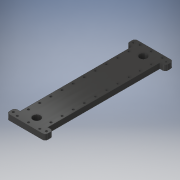
# Autodesk Inventor part: PVCBottom
Saved by Autodesk Inventor 2019.4 (Build 234330000, 330)
## iProperties
Created: 2020-04-27
Part Number: PVCBottom
Material: Generic
Document SubType Name: Modeling
Designer: Ed
Density: 1 g/cm^3
Appearance: Default
Author: Ed
Autodesk Inventor part; units mm, degrees
ref_plane "YZ Plane" through (0, 0, 0) normal (1, 0, 0) x (0, 1, 0)
ref_plane "XZ Plane" through (0, 0, 0) normal (0, 1, 0) x (-1, 0, 0)
ref_plane "XY Plane" through (0, 0, 0) normal (0, 0, 1) x (1, 0, 0)
sketch "Sketch1" plane through (0, 0, 0) normal (0, 1, 0) x (-1, 0, 0)
  line L0 (50.8, 0) -> (52.1295, 0)
  arc A0 (50.8, 16.637) -> (59.7281, 25.5651) centre (50.8, 25.5651) ccw
  arc A1 (59.7281, 25.5651) -> (50.8, 34.4932) centre (50.8, 25.5651) ccw
  arc A2 (50.8, 34.4932) -> (41.8719, 25.5651) centre (50.8, 25.5651) ccw
  arc A3 (41.8719, 25.5651) -> (50.8, 16.637) centre (50.8, 25.5651) ccw
  arc A4 (53.213, 6.35) -> (50.721, 8.7617) centre (50.8, 6.35) ccw
  arc A5 (50.721, 8.7617) -> (50.1755, 8.6808) centre (50.8, 6.35) ccw
  arc A6 (50.1755, 8.6808) -> (48.387, 6.35) centre (50.8, 6.35) ccw
  arc A7 (48.387, 6.35) -> (53.1308, 5.7255) centre (50.8, 6.35) ccw
  arc A8 (53.1308, 5.7255) -> (53.1924, 6.035) centre (50.8, 6.35) ccw
  arc A9 (53.1924, 6.035) -> (53.2078, 6.1922) centre (50.8, 6.35) ccw
  arc A10 (53.2078, 6.1922) -> (53.213, 6.35) centre (50.8, 6.35) ccw
  arc A11 (87.6788, 9.0295) -> (87.7165, 8.8676) centre (90.17, 9.525) ccw
  arc A12 (87.7165, 8.8676) -> (92.71, 9.525) centre (90.17, 9.525) ccw
  arc A13 (92.71, 9.525) -> (87.63, 9.525) centre (90.17, 9.525) ccw
  arc A14 (87.63, 9.525) -> (87.6788, 9.0295) centre (90.17, 9.525) ccw
  arc A15 (77.5292, 8.7623) -> (76.8455, 8.6808) centre (77.47, 6.35) ccw
  arc A16 (76.8455, 8.6808) -> (75.057, 6.35) centre (77.47, 6.35) ccw
  arc A17 (75.057, 6.35) -> (79.883, 6.35) centre (77.47, 6.35) ccw
  arc A18 (79.883, 6.35) -> (79.3353, 7.8808) centre (77.47, 6.35) ccw
  arc A19 (79.3353, 7.8808) -> (77.5292, 8.7623) centre (77.47, 6.35) ccw
  arc A20 (77.6672, 35.3094) -> (76.8455, 35.2352) centre (77.47, 32.9044) ccw
  arc A21 (76.8455, 35.2352) -> (75.057, 32.9044) centre (77.47, 32.9044) ccw
  arc A22 (75.057, 32.9044) -> (77.6278, 30.4966) centre (77.47, 32.9044) ccw
  arc A23 (77.6278, 30.4966) -> (79.5597, 31.6979) centre (77.47, 32.9044) ccw
  arc A24 (79.5597, 31.6979) -> (79.883, 32.9044) centre (77.47, 32.9044) ccw
  arc A25 (79.883, 32.9044) -> (77.9408, 35.2711) centre (77.47, 32.9044) ccw
  arc A26 (77.9408, 35.2711) -> (77.6672, 35.3094) centre (77.47, 32.9044) ccw
  arc A27 (77.5292, 61.8711) -> (76.8455, 61.7896) centre (77.47, 59.4589) ccw
  arc A28 (76.8455, 61.7896) -> (75.057, 59.4589) centre (77.47, 59.4589) ccw
  arc A29 (75.057, 59.4589) -> (76.8455, 57.1281) centre (77.47, 59.4589) ccw
  arc A30 (76.8455, 57.1281) -> (77.391, 57.0472) centre (77.47, 59.4589) ccw
  arc A31 (77.391, 57.0472) -> (79.883, 59.4589) centre (77.47, 59.4589) ccw
  arc A32 (79.883, 59.4589) -> (79.3353, 60.9897) centre (77.47, 59.4589) ccw
  arc A33 (79.3353, 60.9897) -> (77.5292, 61.8711) centre (77.47, 59.4589) ccw
  arc A34 (77.6672, 88.4182) -> (76.8455, 88.3441) centre (77.47, 86.0133) ccw
  arc A35 (76.8455, 88.3441) -> (75.057, 86.0133) centre (77.47, 86.0133) ccw
  arc A36 (75.057, 86.0133) -> (77.6278, 83.6055) centre (77.47, 86.0133) ccw
  arc A37 (77.6278, 83.6055) -> (79.5597, 84.8068) centre (77.47, 86.0133) ccw
  arc A38 (79.5597, 84.8068) -> (79.883, 86.0133) centre (77.47, 86.0133) ccw
  arc A39 (79.883, 86.0133) -> (77.9408, 88.3799) centre (77.47, 86.0133) ccw
  arc A40 (77.9408, 88.3799) -> (77.6672, 88.4182) centre (77.47, 86.0133) ccw
  arc A41 (77.6672, 114.9726) -> (76.8455, 114.8985) centre (77.47, 112.5677) ccw
  arc A42 (76.8455, 114.8985) -> (75.057, 112.5677) centre (77.47, 112.5677) ccw
  arc A43 (75.057, 112.5677) -> (76.8455, 110.2369) centre (77.47, 112.5677) ccw
  arc A44 (76.8455, 110.2369) -> (77.391, 110.156) centre (77.47, 112.5677) ccw
  arc A45 (77.391, 110.156) -> (79.883, 112.5677) centre (77.47, 112.5677) ccw
  arc A46 (79.883, 112.5677) -> (79.6342, 113.635) centre (77.47, 112.5677) ccw
  arc A47 (79.6342, 113.635) -> (77.6672, 114.9726) centre (77.47, 112.5677) ccw
  arc A48 (77.6278, 141.53) -> (76.2635, 141.2119) centre (77.47, 139.1222) ccw
  arc A49 (76.2635, 141.2119) -> (75.057, 139.1222) centre (77.47, 139.1222) ccw
  arc A50 (75.057, 139.1222) -> (77.2335, 136.7208) centre (77.47, 139.1222) ccw
  arc A51 (77.2335, 136.7208) -> (79.1762, 137.4159) centre (77.47, 139.1222) ccw
  arc A52 (79.1762, 137.4159) -> (79.883, 139.1222) centre (77.47, 139.1222) ccw
  arc A53 (79.883, 139.1222) -> (78.0945, 141.4529) centre (77.47, 139.1222) ccw
  arc A54 (78.0945, 141.4529) -> (77.6278, 141.53) centre (77.47, 139.1222) ccw
  arc A55 (77.6278, 168.0844) -> (76.2635, 167.7663) centre (77.47, 165.6766) ccw
  arc A56 (76.2635, 167.7663) -> (75.057, 165.6766) centre (77.47, 165.6766) ccw
  arc A57 (75.057, 165.6766) -> (76.8455, 163.3458) centre (77.47, 165.6766) ccw
  arc A58 (76.8455, 163.3458) -> (77.391, 163.2649) centre (77.47, 165.6766) ccw
  arc A59 (77.391, 163.2649) -> (79.883, 165.6766) centre (77.47, 165.6766) ccw
  arc A60 (79.883, 165.6766) -> (79.5597, 166.8831) centre (77.47, 165.6766) ccw
  arc A61 (79.5597, 166.8831) -> (77.6278, 168.0844) centre (77.47, 165.6766) ccw
  arc A62 (77.6278, 194.6388) -> (76.2635, 194.3207) centre (77.47, 192.231) ccw
  arc A63 (76.2635, 194.3207) -> (75.057, 192.231) centre (77.47, 192.231) ccw
  arc A64 (75.057, 192.231) -> (77.2335, 189.8296) centre (77.47, 192.231) ccw
  arc A65 (77.2335, 189.8296) -> (79.1762, 190.5248) centre (77.47, 192.231) ccw
  arc A66 (79.1762, 190.5248) -> (79.883, 192.231) centre (77.47, 192.231) ccw
  arc A67 (79.883, 192.231) -> (78.0945, 194.5618) centre (77.47, 192.231) ccw
  arc A68 (78.0945, 194.5618) -> (77.6278, 194.6388) centre (77.47, 192.231) ccw
  arc A69 (77.5958, 221.1952) -> (77.4404, 221.1983) centre (77.47, 218.7854) ccw
  arc A70 (77.4404, 221.1983) -> (75.7638, 220.4917) centre (77.47, 218.7854) ccw
  arc A71 (75.7638, 220.4917) -> (75.057, 218.7854) centre (77.47, 218.7854) ccw
  arc A72 (75.057, 218.7854) -> (76.8455, 216.4547) centre (77.47, 218.7854) ccw
  arc A73 (76.8455, 216.4547) -> (77.391, 216.3737) centre (77.47, 218.7854) ccw
  arc A74 (77.391, 216.3737) -> (79.883, 218.7854) centre (77.47, 218.7854) ccw
  arc A75 (79.883, 218.7854) -> (79.7791, 219.4859) centre (77.47, 218.7854) ccw
  arc A76 (79.7791, 219.4859) -> (78.0563, 221.1261) centre (77.47, 218.7854) ccw
  arc A77 (78.0563, 221.1261) -> (77.5958, 221.1952) centre (77.47, 218.7854) ccw
  arc A78 (77.7065, 247.7413) -> (75.7638, 247.0461) centre (77.47, 245.3399) ccw
  arc A79 (75.7638, 247.0461) -> (75.057, 245.3399) centre (77.47, 245.3399) ccw
  arc A80 (75.057, 245.3399) -> (77.2335, 242.9385) centre (77.47, 245.3399) ccw
  arc A81 (77.2335, 242.9385) -> (79.1762, 243.6336) centre (77.47, 245.3399) ccw
  arc A82 (79.1762, 243.6336) -> (79.883, 245.3399) centre (77.47, 245.3399) ccw
  arc A83 (79.883, 245.3399) -> (77.7065, 247.7413) centre (77.47, 245.3399) ccw
  arc A84 (76.8455, 269.5635) -> (77.391, 269.4826) centre (77.47, 271.8943) ccw
  arc A85 (77.391, 269.4826) -> (79.883, 271.8943) centre (77.47, 271.8943) ccw
  arc A86 (79.883, 271.8943) -> (79.7283, 272.7443) centre (77.47, 271.8943) ccw
  arc A87 (79.7283, 272.7443) -> (78.1041, 274.2225) centre (77.47, 271.8943) ccw
  arc A88 (78.1041, 274.2225) -> (77.6364, 274.3016) centre (77.47, 271.8943) ccw
  arc A89 (77.6364, 274.3016) -> (75.1392, 272.5188) centre (77.47, 271.8943) ccw
  arc A90 (75.1392, 272.5188) -> (75.057, 271.8943) centre (77.47, 271.8943) ccw
  arc A91 (75.057, 271.8943) -> (76.8455, 269.5635) centre (77.47, 271.8943) ccw
  arc A92 (13.8835, 8.8676) -> (13.97, 9.525) centre (11.43, 9.525) ccw
  arc A93 (13.97, 9.525) -> (8.89, 9.525) centre (11.43, 9.525) ccw
  arc A94 (8.89, 9.525) -> (13.8835, 8.8676) centre (11.43, 9.525) ccw
  arc A95 (24.13, 8.763) -> (22.7894, 8.3563) centre (24.13, 6.35) ccw
  arc A96 (22.7894, 8.3563) -> (21.717, 6.35) centre (24.13, 6.35) ccw
  arc A97 (21.717, 6.35) -> (26.4608, 5.7255) centre (24.13, 6.35) ccw
  arc A98 (26.4608, 5.7255) -> (26.543, 6.35) centre (24.13, 6.35) ccw
  arc A99 (26.543, 6.35) -> (26.3593, 7.2734) centre (24.13, 6.35) ccw
  arc A100 (26.3593, 7.2734) -> (24.13, 8.763) centre (24.13, 6.35) ccw
  arc A101 (24.2632, 35.3138) -> (24.13, 35.3174) centre (24.13, 32.9044) ccw
  arc A102 (24.13, 35.3174) -> (21.717, 32.9044) centre (24.13, 32.9044) ccw
  arc A103 (21.717, 32.9044) -> (22.7894, 30.8981) centre (24.13, 32.9044) ccw
  arc A104 (22.7894, 30.8981) -> (23.5055, 30.5737) centre (24.13, 32.9044) ccw
  arc A105 (23.5055, 30.5737) -> (24.051, 30.4927) centre (24.13, 32.9044) ccw
  arc A106 (24.051, 30.4927) -> (26.543, 32.9044) centre (24.13, 32.9044) ccw
  arc A107 (26.543, 32.9044) -> (24.6008, 35.2711) centre (24.13, 32.9044) ccw
  arc A108 (24.6008, 35.2711) -> (24.4841, 35.2913) centre (24.13, 32.9044) ccw
  arc A109 (24.4841, 35.2913) -> (24.3075, 35.3109) centre (24.13, 32.9044) ccw
  arc A110 (24.3075, 35.3109) -> (24.2632, 35.3138) centre (24.13, 32.9044) ccw
  arc A111 (24.13, 61.8719) -> (22.7894, 61.4652) centre (24.13, 59.4589) ccw
  arc A112 (22.7894, 61.4652) -> (21.717, 59.4589) centre (24.13, 59.4589) ccw
  arc A113 (21.717, 59.4589) -> (23.5055, 57.1281) centre (24.13, 59.4589) ccw
  arc A114 (23.5055, 57.1281) -> (24.051, 57.0472) centre (24.13, 59.4589) ccw
  arc A115 (24.051, 57.0472) -> (26.543, 59.4589) centre (24.13, 59.4589) ccw
  arc A116 (26.543, 59.4589) -> (24.13, 61.8719) centre (24.13, 59.4589) ccw
  arc A117 (24.2632, 88.4226) -> (24.13, 88.4263) centre (24.13, 86.0133) ccw
  arc A118 (24.13, 88.4263) -> (21.717, 86.0133) centre (24.13, 86.0133) ccw
  arc A119 (21.717, 86.0133) -> (23.5055, 83.6825) centre (24.13, 86.0133) ccw
  arc A120 (23.5055, 83.6825) -> (24.051, 83.6016) centre (24.13, 86.0133) ccw
  arc A121 (24.051, 83.6016) -> (26.543, 86.0133) centre (24.13, 86.0133) ccw
  arc A122 (26.543, 86.0133) -> (24.6008, 88.3799) centre (24.13, 86.0133) ccw
  arc A123 (24.6008, 88.3799) -> (24.4841, 88.4002) centre (24.13, 86.0133) ccw
  arc A124 (24.4841, 88.4002) -> (24.3075, 88.4198) centre (24.13, 86.0133) ccw
  arc A125 (24.3075, 88.4198) -> (24.2632, 88.4226) centre (24.13, 86.0133) ccw
  arc A126 (24.13, 114.9807) -> (22.4238, 114.274) centre (24.13, 112.5677) ccw
  arc A127 (22.4238, 114.274) -> (21.717, 112.5677) centre (24.13, 112.5677) ccw
  arc A128 (21.717, 112.5677) -> (23.5055, 110.2369) centre (24.13, 112.5677) ccw
  arc A129 (23.5055, 110.2369) -> (24.051, 110.156) centre (24.13, 112.5677) ccw
  arc A130 (24.051, 110.156) -> (26.543, 112.5677) centre (24.13, 112.5677) ccw
  arc A131 (26.543, 112.5677) -> (24.13, 114.9807) centre (24.13, 112.5677) ccw
  arc A132 (24.2632, 141.5315) -> (24.13, 141.5352) centre (24.13, 139.1222) ccw
  arc A133 (24.13, 141.5352) -> (21.717, 139.1222) centre (24.13, 139.1222) ccw
  arc A134 (21.717, 139.1222) -> (23.5055, 136.7914) centre (24.13, 139.1222) ccw
  arc A135 (23.5055, 136.7914) -> (24.051, 136.7104) centre (24.13, 139.1222) ccw
  arc A136 (24.051, 136.7104) -> (26.543, 139.1222) centre (24.13, 139.1222) ccw
  arc A137 (26.543, 139.1222) -> (24.6008, 141.4888) centre (24.13, 139.1222) ccw
  arc A138 (24.6008, 141.4888) -> (24.4841, 141.509) centre (24.13, 139.1222) ccw
  arc A139 (24.4841, 141.509) -> (24.3075, 141.5286) centre (24.13, 139.1222) ccw
  arc A140 (24.3075, 141.5286) -> (24.2632, 141.5315) centre (24.13, 139.1222) ccw
  arc A141 (24.13, 168.0896) -> (22.4238, 167.3828) centre (24.13, 165.6766) ccw
  arc A142 (22.4238, 167.3828) -> (21.717, 165.6766) centre (24.13, 165.6766) ccw
  arc A143 (21.717, 165.6766) -> (23.5055, 163.3458) centre (24.13, 165.6766) ccw
  arc A144 (23.5055, 163.3458) -> (24.051, 163.2649) centre (24.13, 165.6766) ccw
  arc A145 (24.051, 163.2649) -> (26.543, 165.6766) centre (24.13, 165.6766) ccw
  arc A146 (26.543, 165.6766) -> (24.13, 168.0896) centre (24.13, 165.6766) ccw
  arc A147 (24.3272, 194.6359) -> (23.5055, 194.5618) centre (24.13, 192.231) ccw
  arc A148 (23.5055, 194.5618) -> (21.717, 192.231) centre (24.13, 192.231) ccw
  arc A149 (21.717, 192.231) -> (23.5055, 189.9002) centre (24.13, 192.231) ccw
  arc A150 (23.5055, 189.9002) -> (24.051, 189.8193) centre (24.13, 192.231) ccw
  arc A151 (24.051, 189.8193) -> (26.543, 192.231) centre (24.13, 192.231) ccw
  arc A152 (26.543, 192.231) -> (24.6008, 194.5976) centre (24.13, 192.231) ccw
  arc A153 (24.6008, 194.5976) -> (24.3272, 194.6359) centre (24.13, 192.231) ccw
  arc A154 (24.051, 221.1971) -> (23.5055, 221.1162) centre (24.13, 218.7854) ccw
  arc A155 (23.5055, 221.1162) -> (22.2156, 220.2544) centre (24.13, 218.7854) ccw
  arc A156 (22.2156, 220.2544) -> (21.717, 218.7854) centre (24.13, 218.7854) ccw
  arc A157 (21.717, 218.7854) -> (23.5055, 216.4547) centre (24.13, 218.7854) ccw
  arc A158 (23.5055, 216.4547) -> (24.051, 216.3737) centre (24.13, 218.7854) ccw
  arc A159 (24.051, 216.3737) -> (26.543, 218.7854) centre (24.13, 218.7854) ccw
  arc A160 (26.543, 218.7854) -> (24.051, 221.1971) centre (24.13, 218.7854) ccw
  arc A161 (24.3272, 247.7448) -> (23.5055, 247.6706) centre (24.13, 245.3399) ccw
  arc A162 (23.5055, 247.6706) -> (21.717, 245.3399) centre (24.13, 245.3399) ccw
  arc A163 (21.717, 245.3399) -> (23.5055, 243.0091) centre (24.13, 245.3399) ccw
  arc A164 (23.5055, 243.0091) -> (24.051, 242.9282) centre (24.13, 245.3399) ccw
  arc A165 (24.051, 242.9282) -> (26.543, 245.3399) centre (24.13, 245.3399) ccw
  arc A166 (26.543, 245.3399) -> (24.6008, 247.7065) centre (24.13, 245.3399) ccw
  arc A167 (24.6008, 247.7065) -> (24.3272, 247.7448) centre (24.13, 245.3399) ccw
  arc A168 (22.9235, 273.984) -> (22.0403, 273.1008) centre (24.13, 271.8943) ccw
  arc A169 (22.0403, 273.1008) -> (21.717, 271.8943) centre (24.13, 271.8943) ccw
  arc A170 (21.717, 271.8943) -> (23.6592, 269.5277) centre (24.13, 271.8943) ccw
  arc A171 (23.6592, 269.5277) -> (24.0116, 269.4842) centre (24.13, 271.8943) ccw
  arc A172 (24.0116, 269.4842) -> (24.13, 269.4813) centre (24.13, 271.8943) ccw
  arc A173 (24.13, 269.4813) -> (26.543, 271.8943) centre (24.13, 271.8943) ccw
  arc A174 (26.543, 271.8943) -> (22.9235, 273.984) centre (24.13, 271.8943) ccw
  arc A175 (13.9212, 295.7705) -> (13.8835, 295.9324) centre (11.43, 295.275) ccw
  arc A176 (13.8835, 295.9324) -> (8.89, 295.275) centre (11.43, 295.275) ccw
  arc A177 (8.89, 295.275) -> (13.97, 295.275) centre (11.43, 295.275) ccw
  arc A178 (13.97, 295.275) -> (13.9212, 295.7705) centre (11.43, 295.275) ccw
  arc A179 (26.3649, 297.539) -> (26.543, 298.4487) centre (24.13, 298.4487) ccw
  arc A180 (26.543, 298.4487) -> (22.1686, 299.8542) centre (24.13, 298.4487) ccw
  arc A181 (22.1686, 299.8542) -> (21.7992, 299.0733) centre (24.13, 298.4487) ccw
  arc A182 (21.7992, 299.0733) -> (21.717, 298.4487) centre (24.13, 298.4487) ccw
  arc A183 (21.717, 298.4487) -> (22.4238, 296.7425) centre (24.13, 298.4487) ccw
  arc A184 (22.4238, 296.7425) -> (23.6592, 296.0821) centre (24.13, 298.4487) ccw
  arc A185 (23.6592, 296.0821) -> (24.1892, 296.0365) centre (24.13, 298.4487) ccw
  arc A186 (24.1892, 296.0365) -> (26.3649, 297.539) centre (24.13, 298.4487) ccw
  arc A187 (50.8, 288.163) -> (41.8719, 279.2349) centre (50.8, 279.2349) ccw
  arc A188 (41.8719, 279.2349) -> (59.7281, 279.2349) centre (50.8, 279.2349) ccw
  arc A189 (59.7281, 279.2349) -> (50.8, 288.163) centre (50.8, 279.2349) ccw
  arc A190 (53.2078, 298.2922) -> (53.213, 298.45) centre (50.8, 298.45) ccw
  arc A191 (53.213, 298.45) -> (48.4692, 299.0745) centre (50.8, 298.45) ccw
  arc A192 (48.4692, 299.0745) -> (48.4076, 298.765) centre (50.8, 298.45) ccw
  arc A193 (48.4076, 298.765) -> (48.3922, 298.6078) centre (50.8, 298.45) ccw
  arc A194 (48.3922, 298.6078) -> (48.3899, 298.5684) centre (50.8, 298.45) ccw
  arc A195 (48.3899, 298.5684) -> (48.387, 298.45) centre (50.8, 298.45) ccw
  arc A196 (48.387, 298.45) -> (53.1308, 297.8255) centre (50.8, 298.45) ccw
  arc A197 (53.1308, 297.8255) -> (53.2078, 298.2922) centre (50.8, 298.45) ccw
  arc A198 (79.8008, 297.8242) -> (79.883, 298.4487) centre (77.47, 298.4487) ccw
  arc A199 (79.883, 298.4487) -> (75.1392, 299.0733) centre (77.47, 298.4487) ccw
  arc A200 (75.1392, 299.0733) -> (75.0776, 298.7637) centre (77.47, 298.4487) ccw
  arc A201 (75.0776, 298.7637) -> (75.057, 298.4487) centre (77.47, 298.4487) ccw
  arc A202 (75.057, 298.4487) -> (75.3803, 297.2422) centre (77.47, 298.4487) ccw
  arc A203 (75.3803, 297.2422) -> (77.3122, 296.0409) centre (77.47, 298.4487) ccw
  arc A204 (77.3122, 296.0409) -> (78.6765, 296.359) centre (77.47, 298.4487) ccw
  arc A205 (78.6765, 296.359) -> (79.8008, 297.8242) centre (77.47, 298.4487) ccw
  arc A206 (92.6883, 294.9435) -> (92.71, 295.275) centre (90.17, 295.275) ccw
  arc A207 (92.71, 295.275) -> (87.63, 295.275) centre (90.17, 295.275) ccw
  arc A208 (87.63, 295.275) -> (92.6235, 294.6176) centre (90.17, 295.275) ccw
  arc A209 (92.6235, 294.6176) -> (92.6883, 294.9435) centre (90.17, 295.275) ccw
  line L1 (50.8, 0) -> (51.2405, 0)
  line L2 (17.78, 0) -> (50.8, 0)
  line L3 (11.43, 0) -> (17.78, 0)
  arc A210 (5.08, 6.35) -> (11.43, 0) centre (11.43, 6.35) ccw
  line L4 (5.08, 9.525) -> (5.08, 6.35)
  line L5 (5.08, 12.7) -> (5.08, 9.525)
  arc A211 (11.43, 19.05) -> (5.08, 12.7) centre (11.43, 12.7) ccw
  line L6 (17.78, 19.05) -> (11.43, 19.05)
  line L7 (17.78, 152.4) -> (17.78, 19.05)
  line L8 (17.78, 285.75) -> (17.78, 152.4)
  line L9 (11.43, 285.75) -> (17.78, 285.75)
  arc A212 (5.08, 292.1) -> (11.43, 285.75) centre (11.43, 292.1) ccw
  line L10 (5.08, 295.275) -> (5.08, 292.1)
  line L11 (5.08, 298.45) -> (5.08, 295.275)
  arc A213 (11.43, 304.8) -> (5.08, 298.45) centre (11.43, 298.45) ccw
  line L12 (17.78, 304.8) -> (11.43, 304.8)
  line L13 (50.8, 304.8) -> (17.78, 304.8)
  line L14 (83.82, 304.8) -> (50.8, 304.8)
  line L15 (90.17, 304.8) -> (83.82, 304.8)
  arc A214 (96.52, 298.45) -> (90.17, 304.8) centre (90.17, 298.45) ccw
  line L16 (96.52, 295.275) -> (96.52, 298.45)
  line L17 (96.52, 292.1) -> (96.52, 295.275)
  arc A215 (90.17, 285.75) -> (96.52, 292.1) centre (90.17, 292.1) ccw
  line L18 (83.82, 285.75) -> (90.17, 285.75)
  line L19 (83.82, 152.4) -> (83.82, 285.75)
  line L20 (83.82, 19.05) -> (83.82, 152.4)
  line L21 (90.17, 19.05) -> (83.82, 19.05)
  arc A216 (96.52, 12.7) -> (90.17, 19.05) centre (90.17, 12.7) ccw
  line L22 (96.52, 9.525) -> (96.52, 12.7)
  line L23 (96.52, 6.35) -> (96.52, 9.525)
  arc A217 (90.17, 0) -> (96.52, 6.35) centre (90.17, 6.35) ccw
  line L24 (83.82, 0) -> (90.17, 0)
  line L25 (52.1295, 0) -> (83.82, 0)
  point P0 (0, 0)
  constraints: 436 point on circle, 218 centre point, 52 end point, 36 equal radius, 36 tangent, 4 perpendicular, 2 parallel, 1 point on line
extrude "Extrusion1" add sketch "Sketch1" along normal blind 12.7
body "Solid1"
